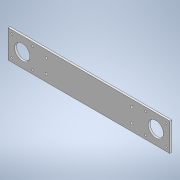
# Autodesk Inventor part: chapa lateral
Saved by Autodesk Inventor 2021 (Build 250183000, 183)
## iProperties
Created: 2022-05-03
Part Number: chapa lateral
Material: Genérico
Document SubType Name: Modeling
Designer: 21155308
Density: 1 g/cm^3
Appearance: Padrão
Author: 21155308
Autodesk Inventor part; units mm, degrees
ref_plane "YZ Plane" through (0, 0, 0) normal (1, 0, 0) x (0, 1, 0)
ref_plane "XZ Plane" through (0, 0, 0) normal (0, 1, 0) x (-1, 0, 0)
ref_plane "XY Plane" through (0, 0, 0) normal (0, 0, 1) x (1, 0, 0)
sketch "Esboço1" plane through (0, 0, 0) normal (0, 0, 1) x (1, 0, 0)
  line L0 (-121, -21) -> (121, -21)
  line L1 (121, -21) -> (121, 21)
  line L2 (121, 21) -> (-121, 21)
  line L3 (-121, 21) -> (-121, -21)
  line L4 (-121, -21) -> (121, 21) construction
  line L5 (121, -21) -> (-121, 21) construction
  point P0 (0, 0)
  dimension "d0" = 242
  dimension "d1" = 42
  constraints: 12 end point, 2 midpoint, 2 parallel, 1 horizontal, 1 perpendicular
  measures "d0" distance of L1.end L2.end
  measures "d1" distance of L2.end L0.start
extrude "Extrusão1" add sketch "Esboço1" along normal blind 3
sketch "Esboço2" plane through (0, 0, 3) normal (0, 0, 1) x (1, 0, 0)
  line L0 (121, 21) -> (-121, 21) projected
  line L1 (-121, 21) -> (-79, 21)
  line L2 (-79, 21) -> (-79, -21)
  line L3 (-79, -21) -> (-121, -21)
  line L4 (-121, -21) -> (-121, 21)
  line L5 (-115.5, -15.5) -> (-84.5, -15.5)
  line L6 (-84.5, -15.5) -> (-84.5, 15.5)
  line L7 (-84.5, 15.5) -> (-115.5, 15.5)
  line L8 (-115.5, 15.5) -> (-115.5, -15.5)
  line L9 (-115.5, -15.5) -> (-84.5, 15.5) construction
  line L10 (-84.5, -15.5) -> (-115.5, 15.5) construction
  point P0 (0, 0)
  point P1 (-100, 0)
  point P2 (-100, 21)
  point P3 (-100, 15.5)
  point P4 (-121, 0)
  point P5 (-115.5, 0)
  dimension "d4" = 42
  dimension "d5" = 42
  dimension "d6" = 31
  dimension "d7" = 31
  constraints: 20 end point, 6 midpoint, 4 parallel, 2 horizontal, 2 perpendicular, 1 horizontal alignment, 1 vertical alignment
  measures "d4" distance of L2.end L3.end
  measures "d5" distance of L1.end L2.end
  measures "d6" distance of L7.end L6.end
  measures "d7" distance of L6.end L5.end
hole "Furo1" at (-115.5, 15.5, 3) at (-84.5, 15.5, 3) at (-84.5, -15.5, 3) at (-115.5, -15.5, 3) direction (0, 0, -1) diameter 3 end through all
hole "Furo2" at (-100, 0, 3) direction (0, 0, -1) diameter 23 end through all
mirror "Espelhamento1" about plane through (0, 0, 0) normal (1, 0, 0) of "Furo1", "Furo2"
sketch "Esboço3" plane through (0, 0, 3) normal (0, 0, 1) x (1, 0, 0)
  circle A0 centre (64, 10.5) radius 1.621 projected
  circle A1 centre (64, -10.5) radius 1.621 projected
  circle A2 centre (-64, 10.5) radius 1.621 projected
  circle A3 centre (-64, -10.5) radius 1.621 projected
  point P0 (0, 0)
hole "Furo3" at (64, -10.5, 3) at (64, 10.5, 3) at (-64, 10.5, 3) at (-64, -10.5, 3) direction (0, 0, -1) diameter 4 end through all
